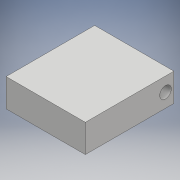
# Autodesk Inventor part: suporteGuiaCentralRetangular
Saved by Autodesk Inventor 2018 (Build 220112000, 112)
## iProperties
Created: 2018-08-22
Part Number: suporteGuiaCentralRetangular
Material: Genérico
Document SubType Name: Modeling
Designer: Georgines
Density: 1 g/cm^3
Appearance: Padrão
Author: Georgines
Autodesk Inventor part; units mm, degrees
ref_plane "YZ Plane" through (0, 0, 0) normal (1, 0, 0) x (0, 1, 0)
ref_plane "XZ Plane" through (0, 0, 0) normal (0, 1, 0) x (-1, 0, 0)
ref_plane "XY Plane" through (0, 0, 0) normal (0, 0, 1) x (1, 0, 0)
sketch "Esboço1" plane through (0, 0, 0) normal (0, 0, 1) x (1, 0, 0)
  circle A0 centre (0, 0) radius 68 construction
  line L0 (-42.5, 47.5) -> (42.5, 47.5)
  line L1 (42.5, -27.5) -> (42.5, -47.5)
  line L2 (42.5, -47.5) -> (-42.5, -47.5)
  line L3 (-42.5, -47.5) -> (-42.5, -27.5)
  line L4 (-42.5, 47.5) -> (42.5, -47.5) construction
  line L5 (42.5, 47.5) -> (-42.5, -47.5) construction
  line L6 (-42.5, -27.5) -> (-42.5, -12.5)
  line L7 (-42.5, -12.5) -> (-42.5, 47.5)
  line L8 (0, 106.3715) -> (0, -163.339) construction
  line L9 (42.5, -27.5) -> (42.5, -12.5)
  line L10 (42.5, -12.5) -> (42.5, 47.5)
  dimension "d0" = 136
  dimension "d1" = 85
  dimension "d2" = 95
  dimension "d13" = 20
  dimension "d14" = 60
  dimension "d15" = 42.5
  constraints: 22 end point, 3 symmetric about line, 2 horizontal, 2 midpoint, 2 parallel, 2 perpendicular, 1 centre point, 1 coincident, 1 vertical
  measures "d0" diameter of A0
  measures "d1" distance of L1.end L2.end
  measures "d2" distance of L5.start L1.end
  measures "d13" distance of L2.end L3.end
  measures "d14" distance of L6.end L0.start
  measures "d15" distance between parallel lines of L8 L7
extrude "Extrusão1" add sketch "Esboço1" along normal mid plane 30
sketch "Esboço2" plane through (42.5, -47.5, 15) normal (1, 0, 0) x (0, 0, -1)
  line L0 (30, 95) -> (0, 95) construction
  line L1 (15, 95) -> (15, 0) construction
  line L2 (30, 0) -> (0, 0) construction
  circle A0 centre (15, 86) radius 6.472 construction
  point P0 (15, 47.5)
  dimension "d5" = 9
  constraints: 2 end point, 2 midpoint, 1 centre point, 1 point on line
  measures "d5" distance from line of A0.centre L0
hole "Furo1" at (42.5, 38.5, 0) direction (-1, 0, 0) diameter 12.5 end through all
